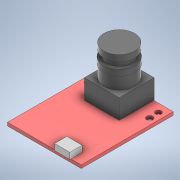
# Autodesk Inventor part: cam001
Saved by Autodesk Inventor 2020 (Build 240168000, 168)
## iProperties
Created: 2024-02-09
Part Number: cam001
Material: Типовые
Document SubType Name: Modeling
Designer: 4s
Density: 1 g/cm^3
Appearance: По умолчанию
Author: 4s
Autodesk Inventor part; units mm, degrees
ref_plane "YZ Plane" through (0, 0, 0) normal (1, 0, 0) x (0, 1, 0)
ref_plane "XZ Plane" through (0, 0, 0) normal (0, 1, 0) x (-1, 0, 0)
ref_plane "XY Plane" through (0, 0, 0) normal (0, 0, 1) x (1, 0, 0)
sketch "Эскиз1" plane through (0, 0, 0) normal (0, 1, 0) x (-1, 0, 0)
  line L0 (-18, -22.5) -> (18, -22.5)
  line L1 (18, -22.5) -> (18, 22.5)
  line L2 (18, 22.5) -> (-18, 22.5)
  line L3 (-18, 22.5) -> (-18, -22.5)
  line L4 (-18, -22.5) -> (18, 22.5) construction
  line L5 (18, -22.5) -> (-18, 22.5) construction
  circle A0 centre (15, -14) radius 1.5
  line L6 (0, -22.5) -> (0, 22.5) construction
  circle A1 centre (-15, -14) radius 1.5
  circle A2 centre (14.75, -18.5) radius 1.4
  circle A3 centre (-14.75, -18.5) radius 1.4
  point P0 (0, 0)
  dimension "d0" = 36
  dimension "d1" = 45
  dimension "d2" = 3
  dimension "d3" = 30
  dimension "d4" = 8.5
  dimension "d5" = 2.8
  dimension "d6" = 29.5
  dimension "d7" = 4
  constraints: 14 end point, 4 centre point, 4 midpoint, 2 parallel, 2 symmetric about line, 1 horizontal, 1 perpendicular, 2 other
  measures "d0" distance of L2.end L1.end
  measures "d1" distance of L1.end L0.end
  measures "d2" diameter of A0
  measures "d3" distance of A0.centre A1.centre
  measures "d4" distance from line of L0 A0.centre
  measures "d5" diameter of A2
  measures "d6" distance of A2.centre A3.centre
  measures "d7" distance from line of L0 A2.centre
extrude "Выдавливание1" add sketch "Эскиз1" against normal blind 1.6
sketch "Эскиз2" plane through (0, 0, 0) normal (0, 1, 0) x (1, 0, 0)
  line L0 (18, 22.5) -> (-18, 22.5) construction
  line L1 (-18, 22.5) -> (-18, -22.5) construction
  line L2 (-18, -22.5) -> (18, -22.5) construction
  line L3 (18, -22.5) -> (18, 22.5) construction
  circle A0 centre (-15, 14) radius 1.5 construction
  circle A1 centre (15, 14) radius 1.5 construction
  circle A2 centre (-14.75, 18.5) radius 1.4 construction
  circle A3 centre (14.75, 18.5) radius 1.4 construction
  line L4 (-15, 14) -> (15, 14) construction
  line L5 (-18, 22.5) -> (18, 22.5) construction
  line L6 (0, 22.5) -> (0, 0) construction
  line L7 (-8.5, 22.6) -> (8.5, 22.6)
  line L8 (8.5, 22.6) -> (8.5, 5.6)
  line L9 (8.5, 5.6) -> (-8.5, 5.6)
  line L10 (-8.5, 5.6) -> (-8.5, 22.6)
  line L11 (-8.5, 5.6) -> (8.5, 22.6) construction
  line L12 (-8.5, 22.6) -> (8.5, 5.6) construction
  point P0 (0, 14.1)
  dimension "d10" = 17
  dimension "d11" = 17
  dimension "d12" = 0.1
  constraints: 16 end point, 3 point on line, 2 horizontal, 2 midpoint, 2 parallel, 1 perpendicular, 1 vertical
  measures "d10" distance of L8.end L9.end
  measures "d11" distance of L7.end L8.end
  measures "d12" distance between parallel lines of L0 L7
extrude "Выдавливание2" add sketch "Эскиз2" along normal blind 9.6
sketch "Эскиз3" plane through (0, 9.6, 0) normal (0, 1, 0) x (1, 0, 0)
  line L0 (8.5, 22.6) -> (-8.5, 22.6) projected
  line L1 (-8.5, 22.6) -> (-8.5, 5.6) projected
  line L2 (-8.5, 5.6) -> (8.5, 5.6) projected
  line L3 (8.5, 5.6) -> (8.5, 22.6) projected
  line L4 (8.5, 22.6) -> (-8.5, 22.6) construction
  line L5 (8.5, 22.6) -> (-8.5, 5.6) construction
  line L6 (-8.5, 22.6) -> (-8.5, 5.6) construction
  line L7 (-8.5, 5.6) -> (8.5, 5.6) construction
  line L8 (-8.5, 22.6) -> (8.5, 5.6) construction
  circle A0 centre (0, 14.1) radius 7.5
  point P0 (0, 0)
  dimension "d15" = 15
  constraints: 4 end point, 1 centre point, 1 midpoint, 1 perpendicular
  measures "d15" diameter of A0
extrude "Выдавливание3" add sketch "Эскиз3" along normal blind 6 contours A0
sketch "Эскиз4" plane through (0, 15.6, -14.1) normal (0, 1, 0) x (1, 0, 0)
  circle A0 centre (0, 0) radius 7.5 projected
  circle A1 centre (0, 0) radius 7.7
  point P0 (0, -14.1)
  dimension "d18" = 15.4
  constraints: 1 centre point, 1 coincident
  measures "d18" diameter of A1
extrude "Выдавливание4" add sketch "Эскиз4" along normal blind 3 contours A0 | A1
sketch "Эскиз5" plane through (0, 18.6, -14.1) normal (0, 1, 0) x (1, 0, 0)
  circle A0 centre (0, 0) radius 7.7 projected
  circle A1 centre (0, 0) radius 6
  point P0 (0, -14.1)
  dimension "d21" = 12
  constraints: 1 centre point, 1 coincident
  measures "d21" diameter of A1
extrude "Выдавливание5" add sketch "Эскиз5" along normal blind 3 contours A1
sketch "Эскиз6" plane through (0, 21.6, -14.1) normal (0, 1, 0) x (1, 0, 0)
  circle A0 centre (0, 0) radius 6 projected
  circle A1 centre (0, 0) radius 7.5
  point P0 (0, -14.1)
  dimension "d24" = 15
  constraints: 1 centre point, 1 coincident
  measures "d24" diameter of A1
extrude "Выдавливание6" add sketch "Эскиз6" along normal blind 3 contours A0 | A1
sketch "Эскиз7" plane through (0, 0, 0) normal (0, 1, 0) x (1, 0, 0)
  line L0 (-8.5, 5.6) -> (-8.5, 22.5) construction
  line L1 (-8.5, 22.5) -> (-18, 22.5) construction
  line L2 (-18, 22.5) -> (-18, -22.5) construction
  line L3 (-18, -22.5) -> (18, -22.5) construction
  line L4 (18, -22.5) -> (18, 22.5) construction
  line L5 (18, 22.5) -> (8.5, 22.5) construction
  line L6 (8.5, 22.5) -> (8.5, 5.6) construction
  line L7 (8.5, 5.6) -> (-8.5, 5.6) construction
  circle A0 centre (-15, 14) radius 1.5 construction
  circle A1 centre (15, 14) radius 1.5 construction
  circle A2 centre (-14.75, 18.5) radius 1.4 construction
  circle A3 centre (14.75, 18.5) radius 1.4 construction
  line L8 (5.5, -17) -> (13, -17)
  line L9 (13, -17) -> (13, -23)
  line L10 (13, -23) -> (5.5, -23)
  line L11 (5.5, -23) -> (5.5, -17)
  point P0 (0, 0)
  dimension "d27" = 7.5
  dimension "d28" = 6
  dimension "d29" = 5
  dimension "d32" = 0.5
  constraints: 8 end point, 2 parallel, 1 horizontal, 1 perpendicular
  measures "d27" distance of L9.end L10.end
  measures "d28" distance of L8.end L9.end
  measures "d29" distance between parallel lines of L4 L9
  measures "d32" distance between parallel lines of L3 L10
extrude "Выдавливание7" add sketch "Эскиз7" along normal blind 3
